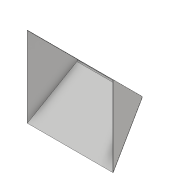
# Autodesk Inventor part: chimneyRoof
Saved by Autodesk Inventor 2017 (Build 210142000, 142)
## iProperties
Created: 2016-12-02
Part Number: chimneyRoof
Material: Generic
Document SubType Name: Sheet Metal
Designer: krosie
Density: 1 g/cm^3
Appearance: Default
Sheet Metal Rule: Default
Author: krosie
Autodesk Inventor part; units mm, degrees
ref_plane "YZ Plane" through (0, 0, 0) normal (1, 0, 0) x (0, 1, 0)
ref_plane "XZ Plane" through (0, 0, 0) normal (0, 1, 0) x (-1, 0, 0)
ref_plane "XY Plane" through (0, 0, 0) normal (0, 0, 1) x (1, 0, 0)
sketch "Sketch1" plane through (0, 0, 0) normal (1, 0, 0) x (0, 1, 0)
  line L0 (-141.4214, 141.4214) -> (-3.5355, 3.5355)
  line L1 (-141.4214, 141.4214) -> (53.5786, 141.4214) construction
  line L2 (-3.5355, -3.5355) -> (-141.4214, -141.4214)
  line L3 (-141.987, -140.8557) -> (-4.6669, -3.5355)
  line L4 (-4.6669, 3.5355) -> (-141.987, 140.8557)
  line L5 (-141.4214, 141.4214) -> (-141.987, 140.8557)
  line L6 (-141.4214, -141.4214) -> (-141.987, -140.8557)
  arc A0 (-4.6669, -3.5355) -> (-4.6669, 3.5355) centre (-8.2024, 0) ccw
  arc A1 (-3.5355, -3.5355) -> (-3.5355, 3.5355) centre (-7.0711, 0) ccw
  point P0 (0, 0)
  point P1 (0, 0)
  point P2 (-1.1314, 0)
  dimension "d0" = 45
  dimension "d1" = 200
  dimension "d2" = 0.8
  dimension "d3" = 0.8
  dimension "d4" = 200
  dimension "d7" = 5
  constraints: 14 end point, 4 point on circle, 4 point on line, 4 tangent, 3 perpendicular, 2 centre point, 1 coincident, 1 equal length, 1 equal radius, 1 horizontal
  measures "d0" angle of L0 L1
  measures "d1" distance of L0.start point (0, 0)
  measures "d2" distance between parallel lines of L0 L4
  measures "d3" distance of L2.end L3.start
  measures "d4" distance of point (0, 0) L2.end
  measures "d7" radius of A0
extrude "Extrusion1" add sketch "Sketch1" along normal blind 300
sketch "Sketch4" plane through (0, 0, 0) normal (0, 0, 1) x (1, 0, 0)
  line L0 (0, -141.4214) -> (0, -3.5355) projected
  line L1 (0, -141.4214) -> (300, -141.4214) projected
  line L2 (300, -3.5355) -> (300, -141.4214) projected
  line L3 (0, -3.5355) -> (300, -3.5355) projected
  line L4 (300, -4.6669) -> (300, -141.987) projected
  line L5 (300, -141.987) -> (261.9547, 0)
  line L6 (300, -141.987) -> (444.3601, -141.987) construction
  line L7 (0, -141.987) -> (145.1381, -141.987) construction
  line L8 (300, -2.5459) -> (300, -141.987)
  line L9 (261.9547, 0) -> (300, 0)
  line L10 (300, -3.5355) -> (300, -141.4214) projected
  line L11 (300, 0) -> (300, -3.5355)
  point P0 (0, 0)
  point P1 (262.6369, -2.5459)
  dimension "d10" = 105
  constraints: 13 end point, 3 horizontal, 1 collinear, 1 perpendicular, 1 point on line
  measures "d10" angle of L6 L5
extrude "Extrusion2" cut sketch "Sketch4" along normal through all both and the other way through all contours L5 L3 L2 L1 | L1 L4 L5 | L5 L9 L11 L8 L3
sketch "Sketch5" plane through (299.8484, -141.4214, -141.4214) normal (0.9659258, 0.258819, 0) x (-0.1798136, 0.6710737, -0.7192546)
  line L0 (-203.4359, 195.6898) -> (-203.4359, 196.504) projected
  line L1 (-5.8996, 202.5394) -> (-203.4359, 195.6898) projected
  ellipse E0 centre (-5.8996, 197.4504) end of major axis (-2.3034, 201.1736) minor radius 5 (-0.8137, 197.6268) -> (-5.8996, 202.5394) ccw projected
  line L2 (-0.8137, -0.0282) -> (-0.8137, 197.6268) projected
  line L3 (0, 0) -> (-0.8137, -0.0282) projected
  line L4 (0, 198.4692) -> (0, 0) projected
  ellipse E1 centre (-5.0859, 198.2929) end of major axis (-8.6822, 194.5697) minor radius 5 (0, 198.4692) -> (-5.0859, 203.3818) ccw projected
  line L5 (-203.4359, 196.504) -> (-5.0859, 203.3818) projected
  line L6 (-0.8137, -0.0282) -> (-203.4359, 195.6898)
  point P0 (47.103, 252.3228)
  constraints: 2 end point, 2 other
extrude "Extrusion3" add sketch "Sketch5" along normal blind 0.8
sketch "Sketch7" plane through (0, 0, 0) normal (0, 0, 1) x (1, 0, 0)
  line L0 (0, -142) -> (38.0488, 0)
  line L1 (0, -142) -> (147.0092, -142) construction
  line L2 (38.0488, 0) -> (0, 0)
  line L3 (0, -3.5355) -> (262.902, -3.5355) projected
  line L4 (0, 0) -> (0, -142)
  dimension "d18" = 75
  constraints: 8 end point, 1 equal length, 1 horizontal, 1 parallel, 1 perpendicular
  measures "d18" angle of L1 L0
extrude "Extrusion4" cut sketch "Sketch7" along normal through all both and the other way through all
sketch "Sketch8" plane through (0.155, -141.4214, 141.4214) normal (-0.9659258, 0.258819, 0) x (0.1798136, 0.6710737, 0.7192546)
  ellipse E0 centre (-5.8996, 197.4504) end of major axis (-2.3034, 201.1736) minor radius 5 (-0.8137, 197.6268) -> (-5.8996, 202.5394) ccw projected
  line L0 (-0.8137, -0.0282) -> (-0.8137, 197.6268) projected
  line L1 (0, 0) -> (-0.8137, -0.0282) projected
  line L2 (0, 198.4692) -> (0, 0) projected
  ellipse E1 centre (-5.0859, 198.2929) end of major axis (-8.6822, 194.5697) minor radius 5 (0, 198.4692) -> (-5.0859, 203.3818) ccw projected
  line L3 (-203.4359, 196.504) -> (-5.0859, 203.3818) projected
  line L4 (-203.4359, 195.6898) -> (-203.4359, 196.504) projected
  line L5 (-5.8996, 202.5394) -> (-203.4359, 195.6898) projected
  line L6 (-0.8137, -0.0282) -> (53.1297, 55.8182) projected
  line L7 (-5.8996, 202.5394) -> (-203.4359, 195.6898) projected
  line L8 (-0.8137, -0.0282) -> (-203.4359, 195.6898)
  point P0 (-6.8417, 196.4751)
  constraints: 2 end point, 2 other
extrude "Extrusion5" add sketch "Sketch8" along normal blind 0.8
equation "\"BendRadius\" = Thickness"
equation "\"BendReliefWidth\" = Thickness"
equation "\"BendReliefDepth\" = 0.5 * Thickness"
equation "\"CornerReliefSize\" = 4 * Thickness"
equation "\"MinimumRemnant\" = 2 * Thickness"
equation "\"TransitionRadius\" = BendRadius"
equation "\"JacobiRadiusSize\" = Thickness"
equation "\"GapSize\" = Thickness"
equation "\"Thickness\" = 0.5"
body "Solid1"
